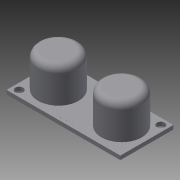
# Autodesk Inventor part: ping
Saved by Autodesk Inventor 2015 (Build 190159000, 159)
## iProperties
Created: 2014-10-24
Part Number: ping
Material: Generic
Document SubType Name: Modeling
Designer: Colin
Density: 1 g/cm^3
Appearance: Default
Author: Colin
Autodesk Inventor part; units mm, degrees
ref_plane "YZ Plane" through (0, 0, 0) normal (1, 0, 0) x (0, 1, 0)
ref_plane "XZ Plane" through (0, 0, 0) normal (0, 1, 0) x (-1, 0, 0)
ref_plane "XY Plane" through (0, 0, 0) normal (0, 0, 1) x (1, 0, 0)
sketch "Sketch1" plane through (0, 0, 0) normal (0, 1, 0) x (-1, 0, 0)
  line L0 (0, 0) -> (-45.72, 0)
  line L1 (-45.72, 0) -> (-45.72, -21.336)
  line L2 (-45.72, -21.336) -> (0, -21.336)
  line L3 (0, -21.336) -> (0, 0)
  circle A0 centre (-2.54, -2.54) radius 1.5875
  circle A1 centre (-43.18, -18.796) radius 1.5875
  line L4 (-22.86, -21.336) -> (-22.86, 0) construction
  circle A2 centre (-22.86, -1.27) radius 0.127
  circle A3 centre (-20.32, -1.27) radius 0.127
  circle A4 centre (-25.4, -1.27) radius 0.127
  dimension "d0" = 21.336
  dimension "d1" = 45.72
  dimension "d2" = 3.175
  dimension "d3" = 2.54
  dimension "d4" = 2.54
  dimension "d5" = 3.175
  dimension "d6" = 2.54
  dimension "d7" = 2.54
  dimension "d9" = 0.254
  dimension "d10" = 0.254
  dimension "d11" = 0.254
  dimension "d12" = 2.54
  dimension "d13" = 2.54
  dimension "d14" = 1.27
  constraints: 10 end point, 5 centre point, 2 midpoint, 2 parallel, 1 horizontal, 1 perpendicular, 1 point on line
  measures "d0" distance of L2.end L0.start
  measures "d1" distance of L1.end L2.end
  measures "d2" diameter of A0
  measures "d3" distance from line of L0 A0.centre
  measures "d4" distance from line of L3 A0.centre
  measures "d5" diameter of A1
  measures "d6" distance from line of L2 A1.centre
  measures "d7" distance from line of L1 A1.centre
  measures "d9" diameter of A2
  measures "d10" diameter of A3
  measures "d11" diameter of A4
  measures "d12" distance of A2.centre A4.centre
  measures "d13" distance of A3.centre A2.centre
  measures "d14" distance from line of L0 A2.centre
extrude "Extrusion1" add sketch "Sketch1" along normal blind 1.57
sketch "Sketch2" plane through (0, 1.57, 0) normal (0, 1, 0) x (1, 0, 0)
  circle A0 centre (10.16, 10.668) radius 8.128
  line L0 (45.72, 21.336) -> (0, 21.336) projected
  line L1 (22.86, 21.336) -> (22.86, 0) construction
  line L2 (0, 0) -> (45.72, 0) projected
  line L3 (0, 21.336) -> (0, 0) projected
  circle A1 centre (35.56, 10.668) radius 8.128
  dimension "d17" = 10.16
  dimension "d18" = 16.256
  dimension "d19" = 10.668
  constraints: 2 centre point, 2 end point, 2 midpoint, 1 symmetric about line, 1 other
  measures "d17" distance from line of L3 A0.centre
  measures "d18" diameter of A0
  measures "d19" distance from line of L0 A0.centre
extrude "Extrusion2" add sketch "Sketch2" along normal blind 13.7
fillet "Fillet1" radius 2.54 1 edges at (2.032, 15.27, -10.668)
fillet "Fillet2" radius 2.54 1 edges at (27.432, 15.27, -10.668)
body "Solid1"
